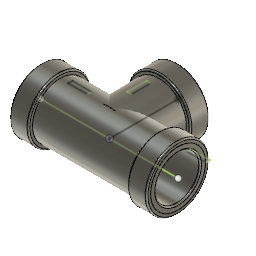
Semana4_Desafio3 v1 (Autodesk Fusion 360 design; units mm, degrees)
Autodesk Fusion 360 part; units mm, degrees
sketch "Sketch2" plane through (0, 0, 0) normal (0, 0, 1) x (1, 0, 0)
  line L0 (-25, 0) -> (25, 0)
  line L1 (0, 0) -> (0, 25)
  dimension "d3" = 25
  constraint horizontal L0
  constraint coincident L1.start origin
  constraint perpendicular L0 L1
  measures "d3" distance of L1.start L1.end
pipe "Pipe1" add diameter 20 wall 2 path "Sketch2" along L0 makes body 1
pipe "Pipe2" add diameter 20 wall 2 path "Sketch2" along L1 separate body makes body 2
pipe "Pipe3" cut diameter 16 path "Sketch2" along L0 bodies 2
pipe "Pipe4" cut diameter 16 path "Sketch2" along L1 bodies 1
sketch "Sketch4" plane through (0, 0, 0) normal (0, 0, 1) x (1, 0, 0)
  line L0 (-25, 10) -> (-18, 10)
  line L1 (-18, 10) -> (-18, 11.5)
  line L2 (-18, 11.5) -> (-25, 11.5)
  line L3 (-25, 11.5) -> (-25, 10)
  line L4 (24.9654, 10) -> (17.9654, 10)
  line L5 (17.9654, 10) -> (17.9654, 11.5)
  line L6 (17.9654, 11.5) -> (24.9833, 11.5)
  line L7 (24.9833, 11.5) -> (24.9654, 10)
  line L8 (-10, 25) -> (-11.5, 25)
  line L9 (-11.5, 25) -> (-11.5, 18)
  line L10 (-11.5, 18) -> (-10, 18)
  line L11 (-10, 25) -> (-10, 18)
  dimension "d26" = 1.5
  dimension "d27" = 7
  dimension "d28" = 7
  dimension "d29" = 1.5
  dimension "d30" = 1.5
  constraint horizontal L0
  constraint perpendicular L0 L1
  constraint perpendicular L1 L2
  constraint perpendicular L0 L3
  constraint perpendicular L3 L4
  constraint perpendicular L4 L5
  constraint perpendicular L5 L6
  constraint equal L1 L5
  constraint collinear L0 L4
  constraint horizontal L8
  constraint perpendicular L8 L9
  constraint perpendicular L9 L10
  measures "d26" distance of L0.end L1.end
  measures "d27" distance of L4.start L4.end
  measures "d28" distance of L1.end L2.end
  measures "d29" distance of L8.start L8.end
  measures "d30" distance of L9.end L10.end
revolve "Revolve3" add sketch "Sketch4" angle 360 about axis through (-25, 0, 0) along (1, 0, 0) contours L4 L5 L6 L7 bodies 1
revolve "Revolve4" add sketch "Sketch4" angle 360 about axis through (-25, 0, 0) along (1, 0, 0) contours L0 L1 L2 L3 bodies 1
revolve "Revolve5" add sketch "Sketch4" angle 360 about axis through (0, 0, 0) along (0, 1, 0) contours L8 L9 L10 L11 bodies 2
fillet "Fillet2" radius 0.5 9 edges at (-25, -7.4586, 2.8929) (-25, -4.1586, 10.7218) (-18, -4.1586, 10.7218) (24.9833, -4.1586, 10.7218) (25, -7.4586, 2.8929) (17.9654, -4.1586, 10.7218) (-7.4586, 25, 2.8929) (-10.7218, 25, 4.1586) (-10.7218, 18, 4.1586) on bodies 1 2
